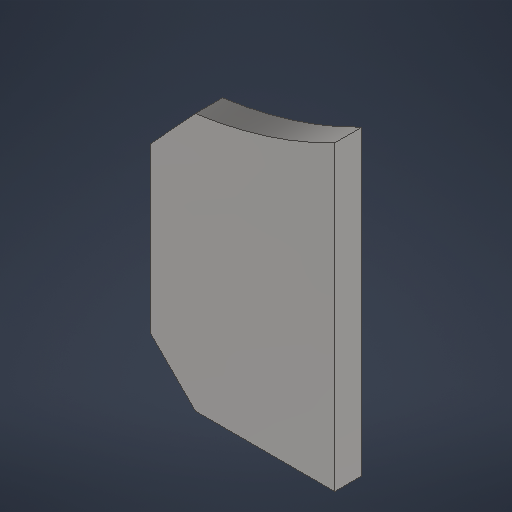
# Autodesk Inventor part: A
Saved by Autodesk Inventor 2025 (Build 290162000, 162)
## iProperties
RuleStatus: InUse
Created: 2024-06-07
Part Number: A
Material: 不鏽鋼
Document SubType Name: Modeling
Designer: a0976
Density: 8 g/cm^3
Appearance: 半拋光
Author: a0976
Autodesk Inventor part; units mm, degrees
ref_plane "YZ Plane" through (0, 0, 0) normal (1, 0, 0) x (0, 1, 0)
ref_plane "XZ Plane" through (0, 0, 0) normal (0, 1, 0) x (-1, 0, 0)
ref_plane "XY Plane" through (0, 0, 0) normal (0, 0, 1) x (1, 0, 0)
sketch "草圖1" plane through (0, 0, 0) normal (0, 0, 1) x (1, 0, 0)
  circle A0 centre (0, 0) radius 136.5
  line L0 (-118.2125, -68.25) -> (-121.8411, -70.345)
  line L1 (118.2125, -68.25) -> (121.8411, -70.345)
  line L2 (-226.66, 0) -> (226.66, 0) projected
  arc A1 (-121.8411, -70.345) -> (121.8411, -70.345) centre (0, 0) ccw
  circle A2 centre (0, 0) radius 132.31
  dimension "d0" = 273
  dimension "d4" = 120
  dimension "d5" = 30
  dimension "d6" = 30
  dimension "d7" = 4.19
  dimension "d12" = 4.19
  constraints: 4 end point, 4 point on circle, 3 centre point, 2 coincident
  measures "d0" diameter of A0
  measures "d4" angle of L1 L0
  measures "d5" angle of L2 L0
  measures "d6" angle of L2 L1
  measures "d7" radial gap between concentric circles of A1 A0
  measures "d12" radial gap between concentric circles of A0 A2
sketch "草圖2" plane through (0, 0, 0) normal (0, 0, 1) x (1, 0, 0)
  line L0 (-44.45, 0) -> (44.45, 0) construction
  line L1 (-65, -236.5) -> (65, -236.5)
  line L2 (0, -136.5) -> (-51.4901, -136.5) construction
  line L3 (0, -140.69) -> (0, -136.45) construction
  line L4 (-65, -224.5) -> (-65, -236.5)
  line L5 (65, -236.5) -> (65, -224.5)
  line L6 (-65, -224.5) -> (-4, -224.5)
  line L7 (4, -224.5) -> (65, -224.5)
  line L8 (-51.4901, -140.69) -> (60.072, -140.69)
  line L9 (-4, -224.5) -> (-4, -140.69)
  line L10 (4, -224.5) -> (4, -140.69)
  arc A0 (-121.8411, -70.345) -> (121.8411, -70.345) centre (0, 0) ccw projected
  circle A1 centre (0, 0) radius 136.5 projected
  point P0 (2.75, -236.5)
  point P1 (-2.75, -236.5)
  point P2 (2.75, -87.55)
  point P3 (-2.75, -87.55)
  dimension "d14" = 100
  dimension "d15" = 130
  dimension "d18" = 12
  dimension "d19" = 8
  dimension "d20" = 8
  dimension "d21" = 12
  dimension "d22" = 130
  constraints: 22 end point, 5 perpendicular, 4 point on line, 3 horizontal, 3 parallel, 1 point on circle, 1 symmetric about line, 1 vertical, 1 vertical alignment, 1 other
  measures "d14" distance from line of L2.start L1
  measures "d15" distance of L1.start L1.end
  measures "d18" distance between parallel lines of L1 L7
  measures "d19" distance between parallel lines of L9 L10
  measures "d20" diameter of L10 L3
  measures "d21" distance between parallel lines of L1 L6
  measures "d22" diameter of L5 L3
sketch "草圖4" plane through (0, 0, 0) normal (0, 0, 1) x (1, 0, 0)
  line L0 (-65, -224.5) -> (-4, -224.5) projected
  line L1 (4, -224.5) -> (65, -224.5) projected
  arc A0 (-121.8411, -70.345) -> (121.8411, -70.345) centre (0, 0) ccw projected
  line L2 (-65, -224.5) -> (-65, -124.7745)
  line L3 (65, -224.5) -> (65, -124.7745)
  line L4 (-4, -224.5) -> (-4, -140.69) projected
  line L5 (4, -224.5) -> (4, -140.69) projected
  line L6 (4, -140.69) -> (4, -140.6331)
  line L7 (-4, -140.69) -> (-4, -140.6331)
  constraints: 8 end point, 4 point on circle, 4 vertical
extrude "擠出6" add sketch "草圖4" along normal mid plane 9 contours L5 L6 A0 L3 L1
chamfer "倒角1" distance 15 angle 45 1 edges at (4, -140.6331, 0)
chamfer "倒角2" distance 15 angle 45 1 edges at (4, -224.5, 0)
equation "\"d12\" = d7"
equation "\"d14\" = Hops"
equation "\"d15\" = Section_buttom_A"
equation "\"d18\" = Section_Top_thick"
equation "\"d19\" = Section_mid_thick"
equation "\"d20\" = Section_mid_thick"
equation "\"d21\" = d18"
equation "\"d22\" = d15"
equation "\"d29\" = Extra_Plate_B"
equation "\"Section_buttom_A\" = 130"
equation "\"Extra_Plate_B\" = 9"
equation "\"Section_mid_thick\" = 8"
equation "\"Section_Top_thick\" = 12"
equation "\"Section_front_gap\" = 35"
equation "\"Section_side_Gap\" = 25"
equation "\"Hops\" = 100"
equation "\"d17\" = Section_Top_thick"
